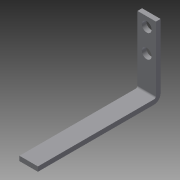
# Autodesk Inventor part: bottom pulley mount
Saved by Autodesk Inventor 2013 (Build 170138000, 138)
## iProperties
Created: 2013-02-07
Part Number: bottom pulley mount
Material: Generic
Document SubType Name: Sheet Metal
Designer: Arpan
Density: 1 g/cm^3
Sheet Metal Rule: Default
Author: Arpan
Autodesk Inventor part; units mm, degrees
ref_plane "YZ Plane" through (0, 0, 0) normal (1, 0, 0) x (0, 1, 0)
ref_plane "XZ Plane" through (0, 0, 0) normal (0, 1, 0) x (-1, 0, 0)
ref_plane "XY Plane" through (0, 0, 0) normal (0, 0, 1) x (1, 0, 0)
sketch "Sketch1" plane through (0, 0, 0) normal (0, 0, 1) x (1, 0, 0)
  line L0 (0, 0) -> (-12.7, 0)
  line L1 (-12.7, 0) -> (-12.7, 44.45)
  line L2 (-12.7, 44.45) -> (0, 44.45)
  line L3 (0, 44.45) -> (0, 0)
  dimension "d0" = 12.7
  dimension "d1" = 44.45
  measures "d0" distance of L0.start L0.end
  measures "d1" distance of L0.end L1.end
extrude "Plate1" add sketch "Sketch1" along normal blind 3.175
sketch "Sketch2" plane through (0, -1.27, 4.445) normal (0, -1, 0) x (1, 0, 0)
  line L0 (-12.7, 0) -> (0, 0)
  line L1 (0, 0) -> (0, 105.3402)
  line L2 (0, 105.3402) -> (-12.7, 105.3402)
  line L3 (-12.7, 105.3402) -> (-12.7, 0)
  constraints: 6 end point, 1 horizontal, 1 perpendicular, 1 vertical
edge flange "Flange1" height 109.7852 angle 90 thickness 3.175 bend radius 1.27 thickness toward (0, -1, 0) relief tear relief width 3.175 relief depth 1.5875 edges at (-6.35, 0, 3.175) wall of the first edge with corners at (-12.7, -1.27, 4.445) (0, -1.27, 4.445) (0, -1.27, 109.7852) (-12.7, -1.27, 109.7852)
bend "Bend1"
corner "Corner1"
sketch "Sketch3" plane through (0, 0, 0) normal (0, 0, -1) x (-1, 0, 0)
  circle A0 centre (6.3516, 38.1) radius 3.3782 projected
  circle A1 centre (6.3516, 22.225) radius 3.3782 projected
extrude "Cut1" cut sketch "Sketch3" against normal blind 3.175
sketch "Sketch4" plane through (-12.7, -4.445, 109.7852) normal (0, -1, 0) x (1, 0, 0)
  line L0 (0, 0) -> (12.7, 0) projected
  line L1 (0, -105.3402) -> (0, 0) projected
  line L2 (6.35, 0) -> (6.35, -12.7)
  circle A0 centre (6.35, -12.7) radius 3.3782
  point P0 (12.7, -109.7852)
  dimension "d15" = 12.7
  dimension "d16" = 6.7564
  constraints: 2 end point, 1 centre point, 1 coincident, 1 midpoint, 1 parallel
  measures "d15" distance of L2.start L2.end
  measures "d16" diameter of A0
extrude "Cut2" cut sketch "Sketch4" against normal blind 3.175
equation "\"d13\" = Thickness"
equation "\"d17\" = Thickness"
equation "\"d3\" = BendReliefWidth"
equation "\"d4\" = BendReliefDepth"
equation "\"d5\" = MinimumRemnant"
equation "\"d6\" = BendRadius"
equation "\"d10\" = CornerReliefSize"
equation "\"d11\" = GapSize"
equation "\"d12\" = JacobiRadiusSize"
equation "\"BendRadius\" = Thickness"
equation "\"BendReliefWidth\" = Thickness"
equation "\"BendReliefDepth\" = 0.5 * Thickness"
equation "\"CornerReliefSize\" = 4 * Thickness"
equation "\"MinimumRemnant\" = 2 * Thickness"
equation "\"TransitionRadius\" = BendRadius"
equation "\"JacobiRadiusSize\" = Thickness"
equation "\"GapSize\" = Thickness"
equation "\"d2\" = BendRadius"
equation "\"Thickness\" = 3.175"
body "Solid1"
